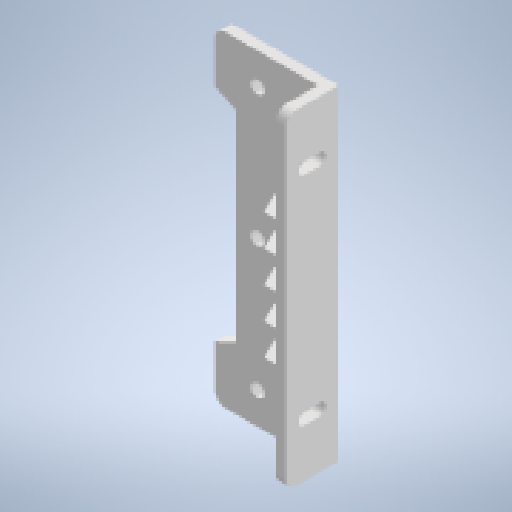
# Autodesk Inventor part: A-07
Saved by Autodesk Inventor 2023 (Build 270158000, 158)
## iProperties
Created: 2022-06-11
Part Number: A-07
Material: Generic
Document SubType Name: Modeling
Designer: kfcs7
Density: 1 g/cm^3
Appearance: Default
Author: kfcs7
Autodesk Inventor part; units mm, degrees
ref_plane "YZ Plane" through (0, 0, 0) normal (1, 0, 0) x (0, 1, 0)
ref_plane "XZ Plane" through (0, 0, 0) normal (0, 1, 0) x (-1, 0, 0)
ref_plane "XY Plane" through (0, 0, 0) normal (0, 0, 1) x (1, 0, 0)
sketch "Sketch1" plane through (0, 0, 0) normal (0, 0, 1) x (1, 0, 0)
  circle A0 centre (0, -25) radius 1.25 construction
  circle A1 centre (0, 25) radius 1.25 construction
  circle A2 centre (0, 0) radius 1.25 construction
  line L0 (6, 28.3) -> (11, 33.3) construction
  line L1 (11, 33.3) -> (11, 41.3) construction
  line L2 (9, 43.3) -> (-9, 43.3) construction
  line L3 (-11, 41.3) -> (-11, 33.3) construction
  line L4 (-11, 33.3) -> (-6, 28.3) construction
  line L5 (-6, 28.3) -> (-6, -28.3) construction
  line L6 (-6, -28.3) -> (-11, -33.3) construction
  line L7 (-11, -33.3) -> (-11, -41.3) construction
  line L8 (-9, -43.3) -> (9, -43.3) construction
  line L9 (11, -41.3) -> (11, -33.3) construction
  line L10 (11, -33.3) -> (6, -28.3) construction
  line L11 (6, -28.3) -> (6, 28.3) construction
  circle A3 centre (-6, -38.3) radius 1.375 construction
  circle A4 centre (6, -38.3) radius 1.375 construction
  circle A5 centre (6, 38.3) radius 1.375 construction
  circle A6 centre (-6, 38.3) radius 1.375 construction
  line L12 (13.5, 47.5) -> (13.5, -47.5) construction
  line L13 (-8, -31) -> (13.5, -31)
  line L14 (13.5, -31) -> (13.5, 31)
  line L15 (13.5, 31) -> (-8, 31)
  line L16 (-8, 31) -> (-8, -31)
  arc A7 (11, 41.3) -> (9, 43.3) centre (9, 41.3) ccw projected
  arc A8 (-9, 43.3) -> (-11, 41.3) centre (-9, 41.3) ccw projected
  arc A9 (-11, -41.3) -> (-9, -43.3) centre (-9, -41.3) ccw projected
  arc A10 (9, -43.3) -> (11, -41.3) centre (9, -41.3) ccw projected
  point P0 (0, 0)
  dimension "d0" = 6
  dimension "d1" = 6
  dimension "d2" = 8
  constraints: 8 end point, 2 parallel, 1 collinear, 1 horizontal, 1 perpendicular
  measures "d0" distance from line of L13 A0.centre
  measures "d1" distance from line of A1.centre L15
  measures "d2" distance from line of A0.centre L16
extrude "Extrusion1" add sketch "Sketch1" along normal blind 10
shell "Shell1" thickness 2 removed faces 4 at (-0.8333, -31, 3.3333) at (-8, 10.3333, 3.3333) at (-0.8333, 10.3333, 10) at (6.3333, 31, 3.3333)
sketch "Sketch2" plane through (11.5, -31, 2) normal (-1, 0, 0) x (0, 0, 1)
  circle A0 centre (3.075, 10.3598) radius 1.25 construction
  circle A1 centre (3.075, 51.6402) radius 1.25 construction
  line L0 (0, 0) -> (0, 62) projected
  line L1 (8, 0) -> (0, 0) projected
  line L2 (8, 62) -> (8, 0) projected
  line L3 (0, 62) -> (8, 62) projected
  line L4 (1.575, 10.3598) -> (4.575, 10.3598) construction
  line L5 (1.575, 9.2348) -> (4.575, 9.2348)
  line L6 (4.575, 11.4848) -> (1.575, 11.4848)
  arc A2 (1.575, 11.4848) -> (1.575, 9.2348) centre (1.575, 10.3598) ccw
  arc A3 (4.575, 9.2348) -> (4.575, 11.4848) centre (4.575, 10.3598) ccw
  line L7 (1.575, 51.6402) -> (4.575, 51.6402) construction
  line L8 (1.575, 50.5152) -> (4.575, 50.5152)
  line L9 (4.575, 52.7652) -> (1.575, 52.7652)
  arc A4 (1.575, 52.7652) -> (1.575, 50.5152) centre (1.575, 51.6402) ccw
  arc A5 (4.575, 50.5152) -> (4.575, 52.7652) centre (4.575, 51.6402) ccw
  line L10 (3.075, 51.6402) -> (6.075, 51.6402) construction
  point P0 (-2, 31)
  dimension "d6" = 1.5
  dimension "d7" = 2.25
  dimension "d8" = 1.5
  dimension "d9" = 0
  dimension "d10" = 2.25
  constraints: 18 end point, 8 point on circle, 8 tangent, 4 centre point, 3 horizontal, 2 midpoint, 2 parallel, 1 collinear
  measures "d6" distance of A0.centre L4.end
  measures "d7" diameter of A3
  measures "d8" distance of L10.start L7.end
  measures "d9" distance between parallel lines of L7 L10
  measures "d10" diameter of A5
extrude "Extrusion2" cut sketch "Sketch2" against normal through all contours A2 L6 A3 L5 | A4 L9 A5 L8
sketch "Sketch3" plane through (-8, 31, 2) normal (0, 0, 1) x (1, 0, 0)
  circle A0 centre (8, -56) radius 1.25 projected
  circle A1 centre (8, -6) radius 1.25 projected
  circle A2 centre (8, -31) radius 1.25 projected
  line L0 (14, -2.7) -> (19, 2.3) projected
  line L1 (19, 2.3) -> (19, 10.3) projected
  line L2 (17, 12.3) -> (-1, 12.3) projected
  line L3 (-3, 10.3) -> (-3, 2.3) projected
  line L4 (-3, 2.3) -> (2, -2.7) projected
  line L5 (2, -2.7) -> (2, -59.3) projected
  line L6 (2, -59.3) -> (-3, -64.3) projected
  line L7 (-3, -64.3) -> (-3, -72.3) projected
  line L8 (-1, -74.3) -> (17, -74.3) projected
  line L9 (19, -72.3) -> (19, -64.3) projected
  line L10 (19, -64.3) -> (14, -59.3) projected
  line L11 (14, -59.3) -> (14, -2.7) projected
  circle A3 centre (2, -69.3) radius 1.375 projected
  circle A4 centre (14, -69.3) radius 1.375 projected
  circle A5 centre (14, 7.3) radius 1.375 projected
  circle A6 centre (2, 7.3) radius 1.375 projected
  arc A7 (19, 10.3) -> (17, 12.3) centre (17, 10.3) ccw projected
  arc A8 (-1, 12.3) -> (-3, 10.3) centre (-1, 10.3) ccw projected
  arc A9 (-3, -72.3) -> (-1, -74.3) centre (-1, -72.3) ccw projected
  arc A10 (17, -74.3) -> (19, -72.3) centre (17, -72.3) ccw projected
  point P0 (8, -31)
extrude "Extrusion3" cut sketch "Sketch3" against normal through all contours A0 | A1 | A2
sketch "Sketch4" plane through (-8, 31, 2) normal (0, 0, 1) x (1, 0, 0)
  line L0 (19.5, -52.7652) -> (19.5, -50.5152) projected
  line L1 (19.5, -11.4848) -> (19.5, -9.2348) projected
  line L2 (19.5, -62) -> (19.5, 0) construction
  line L3 (19.5, -57.1304) -> (15.5, -55.2652)
  line L4 (15.5, -55.2652) -> (15.5, -48.0152)
  line L5 (15.5, -48.0152) -> (19.5, -46.1499)
  line L6 (19.5, -52.7652) -> (15.5, -52.7652) construction
  line L7 (19.5, -50.5152) -> (15.5, -50.5152) construction
  line L8 (19.5, -57.1304) -> (19.5, -46.1499)
  point P0 (8, -31)
  dimension "d15" = 65
  dimension "d16" = 65
  dimension "d18" = 2.5
  dimension "d19" = 2.5
  dimension "d20" = 4
  constraints: 12 end point, 4 point on line, 2 perpendicular, 1 collinear, 1 parallel
  measures "d15" angle of L2 L3
  measures "d16" angle of L2 L5
  measures "d18" distance from line of L3.end L6
  measures "d19" distance from line of L4.end L7
  measures "d20" distance between parallel lines of L0 L4
extrude "Extrusion4" cut sketch "Sketch4" against normal through all
sketch "Sketch5" plane through (-8, 31, 2) normal (0, 0, 1) x (1, 0, 0)
  line L0 (15.5, -48.0152) -> (19.5, -46.1499) projected
  line L1 (19.5, -46.1499) -> (19.5, 0) projected
  line L2 (0, 0) -> (19.5, 0) projected
  line L3 (0, -62) -> (0, 0) projected
  line L4 (19.5, -62) -> (0, -62) projected
  line L5 (19.5, -62) -> (19.5, -57.1304) projected
  line L6 (19.5, -57.1304) -> (15.5, -55.2652) projected
  line L7 (15.5, -55.2652) -> (15.5, -48.0152) projected
  circle A0 centre (8, -6) radius 1.25 projected
  circle A1 centre (8, -31) radius 1.25 projected
  circle A2 centre (8, -56) radius 1.25 projected
  line L8 (0, -52) -> (4, -50.1348)
  line L9 (4, -50.1348) -> (4, -11.8652)
  line L10 (4, -11.8652) -> (0, -10)
  point P0 (8, -31)
  dimension "d25" = 10
  dimension "d26" = 65
  dimension "d27" = 65
  dimension "d28" = 10
  dimension "d29" = 4
  constraints: 6 end point, 2 point on line, 1 vertical
  measures "d25" distance of L2.start L10.end
  measures "d26" angle of L3 L10
  measures "d27" angle of L3 L8
  measures "d28" distance of L3.start L8.start
  measures "d29" distance between parallel lines of L9 L3
extrude "Extrusion5" cut sketch "Sketch5" against normal through all contours L10 L9 L8 L3
mirror "Mirror1" about plane through (0, 0, 0) normal (0, 1, 0) of "Extrusion4"
sketch "Sketch7" plane through (11.5, -31, 10) normal (-1, 0, 0) x (0, 0, 1)
  line L0 (-6.425, 52.7652) -> (-3.425, 52.7652) projected
  arc A0 (-3.425, 50.5152) -> (-3.425, 52.7652) centre (-3.425, 51.6402) ccw projected
  line L1 (-3.425, 50.5152) -> (-6.425, 50.5152) projected
  arc A1 (-6.425, 52.7652) -> (-6.425, 50.5152) centre (-6.425, 51.6402) ccw projected
  line L2 (-6.425, 11.4848) -> (-3.425, 11.4848) projected
  arc A2 (-3.425, 9.2348) -> (-3.425, 11.4848) centre (-3.425, 10.3598) ccw projected
  line L3 (-3.425, 9.2348) -> (-6.425, 9.2348) projected
  arc A3 (-6.425, 11.4848) -> (-6.425, 9.2348) centre (-6.425, 10.3598) ccw projected
  line L4 (-8, 0) -> (-8, 4.8696) projected
  line L5 (0, 0) -> (-8, 0) projected
  line L6 (0, 62) -> (0, 0) projected
  line L7 (-8, 62) -> (0, 62) projected
  line L8 (-8, 57.1304) -> (-8, 62) projected
  line L9 (-8, 57.1304) -> (-10, 57.1304) projected
  line L10 (-10, 46.1499) -> (-10, 57.1304) projected
  line L11 (-8, 46.1499) -> (-10, 46.1499) projected
  line L12 (-8, 15.8501) -> (-8, 46.1499) projected
  line L13 (-8, 15.8501) -> (-10, 15.8501) projected
  line L14 (-10, 4.8696) -> (-10, 15.8501) projected
  line L15 (-8, 4.8696) -> (-10, 4.8696) projected
  line L16 (0, 0) -> (0, 62) projected
  line L17 (0, 31) -> (-8, 31)
  line L18 (0, 32) -> (-8, 32)
  line L19 (0, 30) -> (-8, 30)
  point P0 (-10, 31)
  dimension "d32" = 1
  dimension "d33" = 1
  constraints: 6 end point, 4 point on line, 2 midpoint, 2 perpendicular
  measures "d32" distance between parallel lines of L18 L17
  measures "d33" distance between parallel lines of L17 L19
extrude "Extrusion6" add sketch "Sketch7" along normal blind 6 contours L19 L12 L17 L6 | L17 L12 L18 L6
draft "FaceDraft1" angle 25 pull direction (0, 0, 1) faces at (5.5, 0.3333, 4.6667) fixed edges at (5.5, 0, 2)
pattern_linear "Rectangular Pattern1" count 5 spacing 6 along (0, -1, 0) of "Extrusion6", "FaceDraft1" first direction both ways yes
fillet "Fillet1" radius 2 4 edges at (-8, -31, 1) (-8, 31, 1) (12.5, 31, 10) (12.5, -31, 10)
equation "\"d1\" = d0"
equation "\"d7\" = d10"
equation "\"d16\" = d15"
equation "\"d19\" = d18"
equation "\"d27\" = d26"
equation "\"d28\" = d25"
equation "\"d33\" = d32"
body "Solid1"
